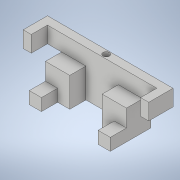
# Autodesk Inventor part: BatteryHolder
Saved by Autodesk Inventor 2020 (Build 240168000, 168)
## iProperties
Created: 2019-06-15
Part Number: BatteryHolder
Material: Generic
Document SubType Name: Modeling
Designer: steele
Density: 1 g/cm^3
Appearance: Default
Author: steele
Autodesk Inventor part; units mm, degrees
ref_plane "YZ Plane" through (0, 0, 0) normal (1, 0, 0) x (0, 1, 0)
ref_plane "XZ Plane" through (0, 0, 0) normal (0, 1, 0) x (-1, 0, 0)
ref_plane "XY Plane" through (0, 0, 0) normal (0, 0, 1) x (1, 0, 0)
sketch "Sketch1" plane through (0, 0, 0) normal (0, 1, 0) x (-1, 0, 0)
  line L0 (63.5, 19.05) -> (-63.5, 19.05)
  line L1 (-63.5, 19.05) -> (-63.5, -19.05)
  line L2 (-63.5, -19.05) -> (63.5, -19.05)
  line L3 (63.5, -19.05) -> (63.5, 19.05)
  line L4 (63.5, 19.05) -> (-63.5, -19.05) construction
  line L5 (-63.5, 19.05) -> (63.5, -19.05) construction
  point P0 (0, 0)
  dimension "baseLength" = 127
  dimension "width" = 38.1
  constraints: 12 end point, 2 midpoint, 2 parallel, 1 horizontal, 1 perpendicular
  measures "baseLength" distance of L0.start L0.end
  measures "width" distance of L1.end L0.end
extrude "Extrusion1" add sketch "Sketch1" along normal blind 46.0375
sketch "Sketch6" plane through (0, 46.0375, 0) normal (0, 1, 0) x (1, 0, 0)
  line L0 (0, 19.05) -> (-98.425, 19.05)
  line L1 (-98.425, 19.05) -> (-98.425, -19.05)
  line L2 (-98.425, -19.05) -> (-85.725, -19.05)
  line L3 (-85.725, -19.05) -> (-85.725, 6.35)
  line L4 (-85.725, 6.35) -> (0, 6.35)
  line L5 (0, 19.05) -> (0, 6.35) construction
  line L6 (0, 19.05) -> (98.425, 19.05)
  line L7 (98.425, 19.05) -> (98.425, -19.05)
  line L8 (98.425, -19.05) -> (85.725, -19.05)
  line L9 (85.725, -19.05) -> (85.725, 6.35)
  line L10 (85.725, 6.35) -> (0, 6.35)
  line L11 (63.5, 19.05) -> (-63.5, 19.05) construction
  line L12 (-63.5, 19.05) -> (63.5, 19.05) construction
  point P0 (0, 0)
  dimension "d29" = 98.425
  dimension "d30" = 38.1
  dimension "d31" = 12.7
  dimension "interiorWidthForBattery" = 25.4
  constraints: 24 end point, 4 symmetric about line, 3 perpendicular, 2 collinear, 2 vertical, 1 horizontal
  measures "d29" distance of L0.start L0.end
  measures "d30" distance of L0.end L1.end
  measures "d31" distance of L1.end L2.end
  measures "interiorWidthForBattery" distance of L2.end L3.end
extrude "Extrusion4" add sketch "Sketch6" along normal blind 25.4
sketch "Sketch7" plane through (-63.5, 0, 19.05) normal (0, 0, 1) x (1, 0, 0)
  line L0 (63.5, 0) -> (63.5, 46.0375) construction
  line L1 (0, 46.0375) -> (127, 46.0375) construction
  line L2 (0, 0) -> (0, 46.0375) projected
  line L3 (0, 0) -> (19.05, 0)
  line L4 (19.05, 0) -> (19.05, 19.05)
  line L5 (19.05, 19.05) -> (0, 19.05)
  line L6 (0, 19.05) -> (0, 0)
  line L7 (127, 0) -> (107.95, 0)
  line L8 (107.95, 0) -> (107.95, 19.05)
  line L9 (107.95, 19.05) -> (127, 19.05)
  line L10 (127, 19.05) -> (127, 0)
  dimension "d35" = 19.05
  dimension "d47" = 19.05
  dimension "d48" = 19.05
  dimension "d49" = 19.05
  constraints: 18 end point, 4 parallel, 2 horizontal, 2 perpendicular, 1 midpoint
  measures "d35" distance of L5.end L4.end
  measures "d47" distance between parallel lines of L5 L3
  measures "d48" distance of L8.end L9.end
  measures "d49" distance of L7.end L8.end
extrude "Extrusion5" add sketch "Sketch7" along normal blind 25.4
sketch "Sketch8" plane through (0, 71.4375, 0) normal (0, 1, 0) x (1, 0, 0)
  line L0 (98.425, 19.05) -> (-98.425, 19.05) projected
  point P0 (0, 0)
  point P1 (0, 12.7)
  dimension "d39" = 6.35
  measures "d39" distance from line of point (0, 12.7) L0
hole "Hole2" at (0, 71.4375, -12.7) direction (0, -1, 0) diameter 10.0838 end through all clearance for "Flat Head Machine Screw (82)" size "3/8" standard "Ansi Unified Screw Threads"
sketch "Sketch9" plane through (-63.5, 46.0375, 19.05) normal (0, 0, 1) x (1, 0, 0)
  line L0 (0, 0) -> (127, 0) construction
  line L1 (63.5, -46.0375) -> (38.1, -46.0375)
  line L2 (38.1, -46.0375) -> (38.1, 0)
  line L3 (38.1, 0) -> (63.5, 0)
  line L4 (63.5, -46.0375) -> (63.5, 0) construction
  line L5 (19.05, -46.0375) -> (107.95, -46.0375) construction
  line L6 (127, 0) -> (0, 0) construction
  line L7 (127, 0) -> (0, 0) construction
  line L8 (63.5, -46.0375) -> (88.9, -46.0375)
  line L9 (88.9, -46.0375) -> (88.9, 0)
  line L10 (88.9, 0) -> (63.5, 0)
  constraints: 18 end point, 6 symmetric about line, 2 horizontal, 2 perpendicular, 2 point on line, 1 parallel
extrude "Extrusion6" cut sketch "Sketch9" against normal blind 25.4
equation "\"d29\" = batterySupportWall + 0.5 * widthForBattery"
equation "\"d30\" = exteriorWidthForBattery"
equation "\"d31\" = batterySupportWall"
equation "\"widthForBattery\" = 171.45"
equation "\"sideLenghtForBattery\" = 25.4"
equation "\"exteriorWidthForBattery\" = 38.1"
equation "\"batterySupportWall\" = 12.7"
body "Solid1"
